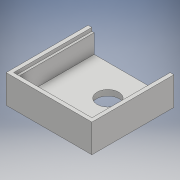
# Autodesk Inventor part: lupa_camera_mount
Saved by Autodesk Inventor 2018 (Build 220112000, 112)
## iProperties
Created: 2017-08-30
Part Number: lupa_camera_mount
Material: Generic
Document SubType Name: Modeling
Designer: matth
Density: 1 g/cm^3
Appearance: Default
Author: matth
Autodesk Inventor part; units mm, degrees
ref_plane "YZ Plane" through (0, 0, 0) normal (1, 0, 0) x (0, 1, 0)
ref_plane "XZ Plane" through (0, 0, 0) normal (0, 1, 0) x (-1, 0, 0)
ref_plane "XY Plane" through (0, 0, 0) normal (0, 0, 1) x (1, 0, 0)
sketch "Sketch1" plane through (0, 0, 0) normal (0, 0, 1) x (1, 0, 0)
  line L0 (-6.959, 4.0688) -> (38.541, 4.0688)
  line L1 (38.541, 4.0688) -> (38.541, -39.4312)
  line L2 (38.541, -39.4312) -> (-6.959, -39.4312)
  line L3 (-6.959, -39.4312) -> (-6.959, 4.0688)
  point P0 (0, 0)
  dimension "d0" = 45.5
  dimension "d1" = 43.5
  constraints: 8 end point, 2 parallel, 1 horizontal, 1 perpendicular
  measures "d0" distance of L1.end L2.end
  measures "d1" distance of L0.end L1.end
extrude "Extrusion1" add sketch "Sketch1" along normal blind 15
sketch "Sketch2" plane through (0, 0, 15) normal (0, 0, 1) x (1, 0, 0)
  line L0 (38.541, 4.0688) -> (-6.959, 4.0688) projected
  line L1 (-4.959, 4.0688) -> (36.541, 4.0688)
  line L2 (36.541, 4.0688) -> (36.541, -37.4312)
  line L3 (36.541, -37.4312) -> (-4.959, -37.4312)
  line L4 (-4.959, -37.4312) -> (-4.959, 4.0688)
  line L5 (-6.959, 4.0688) -> (-6.959, -39.4312) projected
  line L6 (38.541, -39.4312) -> (38.541, 4.0688) projected
  line L7 (-6.959, -39.4312) -> (38.541, -39.4312) projected
  point P0 (0, 0)
  dimension "d4" = 2
  dimension "d5" = 2
  dimension "d6" = 2
  constraints: 8 end point, 2 parallel, 1 horizontal, 1 perpendicular, 1 point on line
  measures "d4" distance between parallel lines of L5 L4
  measures "d5" distance between parallel lines of L6 L2
  measures "d6" distance between parallel lines of L7 L3
extrude "Extrusion2" cut sketch "Sketch2" against normal blind 1.8 contours L2 L3 L4 L0
sketch "Sketch3" plane through (0, 0, 13.2) normal (0, 0, 1) x (1, 0, 0)
  line L0 (-4.959, 4.0688) -> (36.541, 4.0688) projected
  line L1 (-3.759, 4.0688) -> (35.341, 4.0688)
  line L2 (35.341, 4.0688) -> (35.341, -36.2312)
  line L3 (35.341, -36.2312) -> (-3.759, -36.2312)
  line L4 (-3.759, -36.2312) -> (-3.759, 4.0688)
  line L5 (-4.959, -37.4312) -> (-4.959, 4.0688) projected
  line L6 (36.541, -37.4312) -> (-4.959, -37.4312) projected
  line L7 (36.541, 4.0688) -> (36.541, -37.4312) projected
  point P0 (0, 0)
  dimension "d9" = 1.2
  dimension "d10" = 1.2
  dimension "d11" = 1.2
  constraints: 8 end point, 2 parallel, 1 horizontal, 1 perpendicular, 1 point on line
  measures "d9" distance between parallel lines of L5 L4
  measures "d10" distance between parallel lines of L6 L3
  measures "d11" distance between parallel lines of L7 L2
extrude "Extrusion3" cut sketch "Sketch3" against normal blind 10 contours L0 L2 L3 L4
sketch "Sketch4" plane through (0, 0, 0) normal (0, 0, -1) x (-1, 0, 0)
  circle A0 centre (-20.041, -12.4312) radius 6
  line L0 (4.959, -37.4312) -> (4.959, 4.0688) projected
  line L1 (-36.541, -37.4312) -> (4.959, -37.4312) projected
  point P0 (0, 0)
  dimension "d14" = 12
  dimension "d15" = 25
  dimension "d16" = 25
  constraints: 1 centre point
  measures "d14" diameter of A0
  measures "d15" distance from line of L0 A0.centre
  measures "d16" distance from line of L1 A0.centre
sketch "Sketch5" plane through (0, 0, 3.2) normal (0, 0, 1) x (1, 0, 0)
  circle A0 centre (20.041, -12.4312) radius 5.7
  point P0 (0, 0)
  dimension "d17" = 11.4
  constraints: 1 centre point, 1 coincident
  measures "d17" diameter of A0
loft "Loft1" cut profiles "Sketch5", "Sketch4"
body "Solid1"
